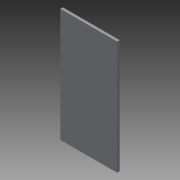
# Autodesk Inventor part: blacha pionowa
Saved by Autodesk Inventor 2015 (Build 190159000, 159)
## iProperties
Created: 2015-05-04
Part Number: blacha pionowa
Material: Ogólny
Document SubType Name: Modeling
Designer: Kuba
Density: 1 g/cm^3
Appearance: Domyślna
Author: Kuba
Autodesk Inventor part; units mm, degrees
ref_plane "YZ Plane" through (0, 0, 0) normal (1, 0, 0) x (0, 1, 0)
ref_plane "XZ Plane" through (0, 0, 0) normal (0, 1, 0) x (-1, 0, 0)
ref_plane "XY Plane" through (0, 0, 0) normal (0, 0, 1) x (1, 0, 0)
sketch "Szkic1" plane through (0, 0, 0) normal (0, 1, 0) x (-1, 0, 0)
  line L0 (-22.5, -45) -> (22.5, -45)
  line L1 (22.5, -45) -> (22.5, 45)
  line L2 (22.5, 45) -> (-22.5, 45)
  line L3 (-22.5, 45) -> (-22.5, -45)
  line L4 (-22.5, -45) -> (22.5, 45) construction
  line L5 (22.5, -45) -> (-22.5, 45) construction
  point P0 (0, 0)
  dimension "d0" = 45
  dimension "d1" = 90
  constraints: 12 end point, 2 midpoint, 2 parallel, 1 horizontal, 1 perpendicular
  measures "d0" distance of L2.end L1.end
  measures "d1" distance of L1.end L0.end
extrude "Wyciągnięcie proste1" add sketch "Szkic1" along normal blind 2
sketch "Szkic2" plane through (0, 2, 0) normal (0, 1, 0) x (1, 0, 0)
  line L0 (11.5, 3.5) -> (18.5, 3.5) projected
  line L1 (18.5, 3.5) -> (18.5, 35.5) projected
  line L2 (18.5, 35.5) -> (-20.5, 35.5) projected
  line L3 (-20.5, 35.5) -> (-20.5, -35.5) projected
  line L4 (-20.5, -35.5) -> (18.5, -35.5) projected
  line L5 (18.5, -35.5) -> (18.5, -26.5) projected
  line L6 (18.5, -26.5) -> (11.5, -26.5) projected
  line L7 (11.5, -26.5) -> (11.5, 3.5) projected
  circle A0 centre (6, 0) radius 1.5 projected
  circle A1 centre (14, 31.5) radius 1.5 projected
  circle A2 centre (-16, -31.5) radius 1.5 projected
  circle A3 centre (-16, 31.5) radius 1.5 projected
  circle A4 centre (14, -31.5) radius 1.5 projected
  circle A5 centre (-16, 0) radius 1.5 projected
  point P0 (0, 0)
hole "Otwór1" at (14, 2, -31.5) at (6, 2, 0) at (14, 2, 31.5) at (-16, 2, 31.5) at (-16, 2, 0) at (-16, 2, -31.5) direction (0, -1, 0) diameter 3.5 end through all
